Autodesk Fusion 360 part; units mm, degrees
(part 2 of 2)
  arc A185 (36.111, 28.317) -> (36.111, 28.9662) centre (36.111, 28.6416) ccw
  line L756 (10.3187, 51.2288) -> (10.3187, 43.6088)
  line L757 (11.5888, 43.6088) -> (11.5888, 42.8468)
  line L758 (34.6508, 29.4855) -> (34.9754, 29.4855)
  line L759 (34.9754, 28.8363) -> (34.6508, 28.8363)
  arc A186 (9.6537, 49.5828) -> (9.0045, 49.5828) centre (9.3291, 49.5828) ccw
  line L760 (35.4013, 26.035) -> (35.4013, 26.797)
  line L761 (13.335, 43.6088) -> (15.875, 43.6088)
  line L762 (9.5238, 50.7833) -> (9.5238, 50.3938)
  line L763 (13.335, 51.2288) -> (13.335, 43.6088)
  line L764 (14.605, 43.6088) -> (14.605, 42.8468)
  line L765 (15.875, 51.2288) -> (13.335, 51.2288)
  line L766 (10.173, 49.9073) -> (9.6537, 49.6477)
  line L767 (15.875, 43.6088) -> (15.875, 51.2288)
  arc A187 (42.1887, 7.893) -> (41.8275, 7.5318) centre (42.1887, 7.5318) ccw
  line L768 (38.2999, 28.1745) -> (38.0403, 28.6938)
  arc A188 (16.67, 43.5828) -> (16.0208, 43.5828) centre (16.3454, 43.5828) ccw
  line L769 (35.7864, 29.4855) -> (36.1759, 29.4855)
  arc A189 (9.7835, 51.0429) -> (9.5239, 50.7833) centre (9.7835, 50.7833) ccw
  arc A190 (36.1759, 28.9662) -> (36.1759, 29.4854) centre (36.1759, 29.2258) ccw
  arc A191 (37.9754, 28.6938) -> (37.9754, 29.343) centre (37.9754, 29.0184) ccw
  line L770 (36.6713, 26.035) -> (34.1313, 26.035)
  line L771 (12.8588, 51.2288) -> (10.3187, 51.2288)
  arc A192 (34.9754, 28.8363) -> (34.9754, 29.4855) centre (34.9754, 29.1609) ccw
  line L772 (39.5288, 26.035) -> (36.9888, 26.035)
  arc A193 (7.0485, 20.1406) -> (7.6355, 20.2761) centre (7.0485, 21.4802) ccw
  line L773 (9.0926, 39.3417) -> (9.0926, 38.1733)
  line L774 (6.5583, 39.3417) -> (7.2074, 39.3417)
  line L775 (42.3863, 26.035) -> (39.8463, 26.035)
  line L776 (33.492, 39.5042) -> (34.1412, 39.5042)
  arc A194 (40.4754, 28.5513) -> (40.4754, 29.2005) centre (40.4754, 28.8759) ccw
  line L777 (33.8166, 38.3358) -> (33.8166, 39.5042)
  line L778 (41.1163, 18.415) -> (41.1163, 17.653)
  arc A195 (8.8801, 47.012) -> (8.8801, 47.6612) centre (8.8801, 47.3366) ccw
  line L779 (17.1892, 43.2582) -> (16.0208, 43.2582)
  arc A196 (16.7997, 45.0429) -> (16.5401, 44.7833) centre (16.7997, 44.7833) ccw
  line L780 (8.9451, 47.6612) -> (8.6854, 47.6612)
  line L781 (34.6139, 38.3358) -> (34.6139, 39.5042)
  line L782 (8.0047, 38.6926) -> (7.6801, 38.6926)
  arc A197 (16.8646, 44.3938) -> (16.8646, 45.043) centre (16.8646, 44.7184) ccw
  line L783 (40.1508, 28.0321) -> (40.1508, 29.2005)
  line L784 (6.8829, 38.1733) -> (6.8829, 39.3417)
  arc A198 (36.351, 39.2121) -> (36.0589, 39.5042) centre (36.0589, 39.2121) ccw
  arc A199 (7.7922, 47.5313) -> (7.7922, 48.1805) centre (7.7922, 47.8559) ccw
  line L785 (34.9384, 38.8551) -> (34.6139, 38.8551)
  line L786 (41.2864, 29.0706) -> (41.2864, 29.2005)
  line L787 (7.7922, 47.5313) -> (7.4676, 47.5313)
  line L788 (16.6699, 43.5828) -> (16.6699, 43.2582)
  line L789 (36.2536, 38.9849) -> (35.7018, 38.3358)
  line L790 (8.5556, 48.1805) -> (8.9451, 48.1805)
  line L791 (8.7681, 38.1733) -> (9.4172, 38.1733)
  line L792 (10.173, 50.3938) -> (10.173, 50.7833)
  line L793 (7.6801, 39.3417) -> (8.0047, 39.3417)
  line L794 (11.5888, 51.2288) -> (11.5888, 51.9908)
  line L795 (39.8463, 26.035) -> (39.8463, 18.415)
  circle A200 centre (8.0475, 36.6938) radius 1.27
  line L796 (40.1508, 29.2005) -> (40.4754, 29.2005)
  line L797 (42.3863, 18.415) -> (42.3863, 26.035)
  line L798 (39.8463, 18.415) -> (42.3863, 18.415)
  circle A201 centre (8.0412, 45.3738) radius 1.27
  line L799 (6.6704, 47.0121) -> (6.6704, 48.1805)
  line L800 (7.4676, 48.1805) -> (7.7922, 48.1805)
  line L801 (6.3458, 48.1805) -> (6.9949, 48.1805)
  line L802 (40.4754, 28.5513) -> (40.1508, 28.5513)
  arc A202 (8.0047, 38.6925) -> (8.0047, 39.3417) centre (8.0047, 39.0171) ccw
  line L803 (17.1892, 43.9073) -> (16.6699, 43.6477)
  line L804 (41.2864, 29.2005) -> (41.9355, 29.2005)
  line L805 (41.9355, 29.2005) -> (41.611, 28.0321)
  line L806 (8.7681, 39.0821) -> (9.0926, 39.3417)
  line L807 (7.6801, 38.1733) -> (7.6801, 39.3417)
  line L808 (10.173, 49.2582) -> (9.0046, 49.2582)
  line L809 (41.1163, 26.035) -> (41.1163, 26.797)
  arc A203 (16.0208, 44.9131) -> (16.5401, 44.3938) centre (16.5401, 44.9131) ccw
  line L810 (40.7999, 28.0321) -> (40.5403, 28.5513)
  circle A204 centre (35.0288, 36.6975) radius 1.27
  dimension "d1" = 53
  dimension "d2" = 55
  measures "d1" distance of L347 L361
  measures "d2" distance of A48.start A52.end
ref_plane "Arbeitsebene3" through (26.5, 27.5, -3) normal (0, 0, 1) x (1, 0, 0)
sketch "Skizze2" plane through (26.5, 27.5, -3) normal (0, 0, 1) x (1, 0, 0)
  circle A0 centre (-22.5, 23.5) radius 1.5875
  line L0 (25.5, 27.5) -> (-25.5, 27.5)
  arc A1 (-25.5, 27.5) -> (-26.5, 26.5) centre (-25.5, 26.5) ccw
  line L1 (-26.5, -26.5) -> (-26.5, 26.5)
  line L2 (-25.5, -27.5) -> (25.5, -27.5)
  arc A2 (-26.5, -26.5) -> (-25.5, -27.5) centre (-25.5, -26.5) ccw
  arc A3 (25.5, -27.5) -> (26.5, -26.5) centre (25.5, -26.5) ccw
  line L3 (26.5, -26.5) -> (26.5, 26.5)
  arc A4 (26.5, 26.5) -> (25.5, 27.5) centre (25.5, 26.5) ccw
  circle A5 centre (22.5, 23.5) radius 3.1
  circle A6 centre (22.5, 23.5) radius 1.5875
  circle A7 centre (-22.5, 23.5) radius 3.1
  line L4 (-36, -27.5) -> (36, -27.5)
  line L5 (36.5, -27) -> (36.5, 28.5)
  line L6 (34.5, 30.5) -> (-34.5, 30.5)
  line L7 (-36.5, 28.5) -> (-36.5, -27)
  arc A8 (-34.5, 30.5) -> (-36.5, 28.5) centre (-34.5, 28.5) ccw
  arc A9 (36.5, 28.5) -> (34.5, 30.5) centre (34.5, 28.5) ccw
  arc A10 (-36.5, -27) -> (-36, -27.5) centre (-36, -27) ccw
  arc A11 (36, -27.5) -> (36.5, -27) centre (36, -27) ccw
  line L8 (-33.5, -25.5) -> (33.5, -25.5)
  line L9 (34.5, -24.5) -> (34.5, 27.5)
  line L10 (33.5, 28.5) -> (-33.5, 28.5)
  line L11 (-34.5, 27.5) -> (-34.5, -24.5)
  arc A12 (-33.5, 28.5) -> (-34.5, 27.5) centre (-33.5, 27.5) ccw
  arc A13 (-34.5, -24.5) -> (-33.5, -25.5) centre (-33.5, -24.5) ccw
  arc A14 (33.5, -25.5) -> (34.5, -24.5) centre (33.5, -24.5) ccw
  arc A15 (34.5, 27.5) -> (33.5, 28.5) centre (33.5, 27.5) ccw
  line L12 (-27, -25.5) -> (-27, -27.5)
  line L13 (27, -25.5) -> (27, -27.5)
  line L14 (35.3, -24.5) -> (35.3, 27.5)
  arc A16 (35.3, 27.5) -> (33.5, 29.3) centre (33.5, 27.5) ccw
  line L15 (33.5, 29.3) -> (-33.5, 29.3)
  arc A17 (-33.5, 29.3) -> (-35.3, 27.5) centre (-33.5, 27.5) ccw
  line L16 (-35.3, 27.5) -> (-35.3, -24.5)
  arc A18 (-35.3, -24.5) -> (-33.5, -26.3) centre (-33.5, -24.5) ccw
  line L17 (-33.5, -26.3) -> (33.5, -26.3)
  arc A19 (33.5, -26.3) -> (35.3, -24.5) centre (33.5, -24.5) ccw
  circle A20 centre (-22.5, 23.5) radius 4
  circle A21 centre (22.5, 23.5) radius 4
  circle A22 centre (30.75, -19.5) radius 1.75
  circle A23 centre (30.75, -19.5) radius 3.75
  circle A24 centre (-30.75, -19.5) radius 1.75
  circle A25 centre (-30.75, -19.5) radius 3.75
  line L18 (24.5, -5) -> (28.5, -5)
  line L19 (28.5, -5) -> (28.5, -7)
  line L20 (28.5, -7) -> (24.5, -7)
  line L21 (24.5, -7) -> (24.5, -5)
  line L22 (27, -5) -> (27, -7)
  line L23 (-28.5, -5) -> (-24.5, -5)
  line L24 (-24.5, -5) -> (-24.5, -7)
  line L25 (-24.5, -7) -> (-28.5, -7)
  line L26 (-28.5, -7) -> (-28.5, -5)
  line L27 (-27, -5) -> (-27, -7)
  point P0 (-23.84, -27.5)
  point P1 (-26.5, -27.5)
  point P2 (-26.5, -26.5)
  dimension "d6" = 2
  dimension "d7" = 2
  dimension "d8" = 3
  dimension "d9" = 10
  dimension "d10" = 10
  dimension "d11" = 0.5
  dimension "d12" = 0.5
  dimension "d14" = 1
  dimension "d15" = 1
  dimension "d16" = 1
  dimension "d17" = 2
  dimension "d18" = 2
  dimension "d19" = 2
  dimension "d20" = 1
  dimension "d21" = 2
  dimension "d22" = 0.5
  dimension "d23" = 0.5
  dimension "d24" = 0.8
  dimension "d25" = 8
  dimension "d26" = 8
  dimension "d27" = 3.5
  dimension "d28" = 7.5
  dimension "d29" = 3.75
  dimension "d30" = 6
  dimension "d31" = 3.5
  dimension "d32" = 7.5
  dimension "d33" = 3.75
  dimension "d34" = 6
  dimension "d35" = 4
  dimension "d36" = 1.5
  dimension "d37" = 2
  dimension "d38" = 2
  dimension "d39" = 18.5
  dimension "d40" = 2
  dimension "d41" = 4
  dimension "d42" = 18.5
  dimension "d43" = 2
  dimension "d44" = 1.5
  constraint parallel L2 L4
  constraint perpendicular L4 L5
  constraint perpendicular L5 L6
  constraint perpendicular L4 L7
  constraint tangent L6 A8
  constraint tangent L7 A8
  constraint tangent L5 A9
  constraint tangent L6 A9
  constraint collinear L2 L4
  constraint tangent L4 A10
  constraint tangent L7 A10
  constraint tangent L4 A11
  constraint tangent L5 A11
  constraint parallel L4 L8
  constraint parallel L5 L9
  constraint parallel L6 L10
  constraint parallel L7 L11
  constraint tangent L10 A12
  constraint tangent L11 A12
  constraint tangent L8 A13
  constraint tangent L11 A13
  constraint tangent L8 A14
  constraint tangent L9 A14
  constraint tangent L9 A15
  constraint tangent L10 A15
  constraint coincident L8 L12.start
  constraint coincident L4 L12.end
  constraint perpendicular L4 L12
  constraint coincident L8 L13.start
  constraint coincident L4 L13.end
  constraint perpendicular L4 L13
  constraint concentric A7 A20
  constraint concentric A5 A21
  constraint concentric A22 A23
  constraint concentric A24 A25
  constraint horizontal L18
  constraint vertical L19
  constraint horizontal L20
  constraint vertical L21
  constraint coincident L18 L22.start
  constraint coincident L20 L22.end
  constraint perpendicular L20 L22
  constraint horizontal L23
  constraint vertical L24
  constraint horizontal L25
  constraint vertical L26
  constraint coincident L23 L27.start
  constraint coincident L25 L27.end
  constraint perpendicular L25 L27
  measures "d6" radius of A8
  measures "d7" radius of A9
  measures "d8" distance of L0 L6
  measures "d9" distance of L1 L7
  measures "d10" distance of L3 L5
  measures "d11" radius of A10
  measures "d12" radius of A11
  measures "d14" radius of A12
  measures "d15" radius of A13
  measures "d16" radius of A14
  measures "d17" distance of L7 L11
  measures "d18" distance of L6 L10
  measures "d19" distance of L5 L9
  measures "d20" radius of A15
  measures "d21" distance of L4 L8
  measures "d22" distance of L1 L12
  measures "d23" distance of L3 L13
  measures "d25" diameter of A20
  measures "d26" diameter of A21
  measures "d27" diameter of A22
  measures "d28" diameter of A23
  measures "d29" distance of L9 A22.centre
  measures "d30" distance of L8 A22.centre
  measures "d31" diameter of A24
  measures "d32" diameter of A25
  measures "d33" distance of L11 A24.centre
  measures "d34" distance of L8 A24.centre
  measures "d35" distance of L18.start L18.end
  measures "d36" distance of L19.end L22.end
  measures "d37" distance of L18.start L20.end
  measures "d38" distance of L3 L19.end
  measures "d39" distance of L8 L19.end
  measures "d40" distance of L23.end L24.end
  measures "d41" distance of L24.end L25.end
  measures "d42" distance of L8 L25.end
  measures "d43" distance of L1 L23.start
  measures "d44" distance of L26 L27
extrude "Extrusion1" add sketch "Skizze2" against normal blind 2 contours A0 | L0 L3 A4 A21 | A23 | A25 | L0 A1 L1 L3 A4 L8 L9 L10 L11 A12 A13 A14 A15 L18 L19 L20 L23 L25 L26 | L0 L1 L3 L8 A20 A21 L18 L20 L21 L23 L24 L25 | A21 | L0 A1 L1 A20 | A20 | L3 L18 L20 L22 | L3 L18 L20 L21 | L1 L23 L24 L25 | L1 L23 L25 L27 | L18 L19 L20 L22 | L23 L25 L26 L27 | L3 L8 L13 L17 | L1 L3 L8 L17 | L1 L8 L12 L17 | A3 L3 L4 L13 L17 | L1 L2 A2 A3 L3 L4 L17 | L8 L9 L10 L11 A12 A13 A14 A15 L12 L13 L14 A16 L15 A17 L16 A18 L17 A19 | L1 A2 L4 L12 L17 | L4 L5 L6 L7 A8 A9 A10 A11 L12 L13 L14 A16 L15 A17 L16 A18 L17 A19 | A5 | A6 | A7 | A22 | A24 makes body 1
extrude "Extrusion2" add sketch "Skizze2" along normal blind 3 contours A21 | A20 | L3 L18 L20 L22 | L3 L18 L20 L21 | L1 L23 L24 L25 | L1 L23 L25 L27 | L18 L19 L20 L22 | L23 L25 L26 L27 | A5 | A7 bodies 1
chamfer "Fase1" distance 1 angle 45 2 edges at (0.2707, 49.5535, 0) (45.2707, 49.5535, 0) on bodies 1
extrude "Extrusion3" add sketch "Skizze2" along normal blind 4.6 contours L23 L25 L26 L27 bodies 1
extrude "Extrusion4" cut sketch "Skizze2" along normal blind 4.6 contours L18 L19 L20 L22 bodies 1
extrude "Extrusion5" add sketch "Skizze2" along normal blind 4.6 contours L18 L19 L20 L22 bodies 1
extrude "Extrusion6" add sketch "Skizze2" along normal blind 4.6 contours A23 | A25 bodies 1
extrude "Extrusion7" add sketch "Skizze2" along normal blind 2 contours L3 L8 L13 L17 | L1 L3 L8 L17 | L1 L8 L12 L17 | A3 L3 L4 L13 L17 | L1 L2 A2 A3 L3 L4 L17 | L1 A2 L4 L12 L17 bodies 1
extrude "Extrusion8" add sketch "Skizze2" along normal blind 9 contours L4 L5 L6 L7 A8 A9 A10 A11 L12 L13 L14 A16 L15 A17 L16 A18 L17 A19 bodies 1
extrude "Extrusion9" add sketch "Skizze2" along normal blind 10 separate body contours L8 L9 L10 L11 A12 A13 A14 A15 L12 L13 L14 A16 L15 A17 L16 A18 L17 A19 makes body 2
sketch "Skizze3" plane through (0, 0, -5) normal (0, 0, -1) x (1, 0, 0)
  arc A0 (63, -0.5) -> (62.5, 0) centre (62.5, -0.5) ccw
  line L0 (62.5, 0) -> (-9.5, 0)
  arc A1 (-9.5, 0) -> (-10, -0.5) centre (-9.5, -0.5) ccw
  line L1 (-10, -0.5) -> (-10, -56)
  arc A2 (-10, -56) -> (-8, -58) centre (-8, -56) ccw
  line L2 (-8, -58) -> (61, -58)
  arc A3 (61, -58) -> (63, -56) centre (61, -56) ccw
  line L3 (63, -56) -> (63, -0.5)
  circle A4 centre (-4.25, -8) radius 1.75
  circle A5 centre (57.25, -8) radius 1.75
  circle A6 centre (49, -51) radius 1.5875
  circle A7 centre (4, -51) radius 1.5875
  circle A8 centre (-4.25, -8) radius 3
  circle A9 centre (57.25, -8) radius 3
  circle A10 centre (49, -51) radius 3
  circle A11 centre (4, -51) radius 3
  dimension "d64" = 6
  dimension "d65" = 6
  dimension "d66" = 6
  dimension "d67" = 6
  constraint concentric A4 A8
  constraint concentric A5 A9
  constraint concentric A6 A10
  constraint concentric A7 A11
  measures "d64" diameter of A8
  measures "d65" diameter of A9
  measures "d66" diameter of A10
  measures "d67" diameter of A11
extrude "Extrusion10" cut sketch "Skizze3" against normal blind 2 contours A4 | A5 | A6 | A7 bodies 1
extrude "Extrusion11" cut sketch "Skizze3" against normal blind 1.5 contours A8 | A9 | A10 | A11 bodies 1
fillet "Abrundung1" radius 2 8 edges at (-10, 28.25, -5) (-9.4142, 57.4142, -5) (26.5, 58, -5) (62.4142, 57.4142, -5) (63, 28.25, -5) (62.8536, 0.1464, -5) (26.5, 0, -5) (-9.8536, 0.1464, -5) on bodies 1
fillet "Abrundung2" radius 1 4 edges at (0, 22.5, -3) (2, 21.5, -3) (0, 20.5, -3) (-2, 21.5, -3) on bodies 1
fillet "Abrundung3" radius 1 4 edges at (53, 20.5, -3) (51, 21.5, -3) (53, 22.5, -3) (55, 21.5, -3) on bodies 1
combine "Kombinieren1" operation add target body 1 tool bodies 2
ref_plane "Arbeitsebene4" through (26.5, 27.5, 9.6) normal (0, 0, 1) x (1, 0, 0)
sketch "Skizze4" plane through (26.5, 27.5, 9.6) normal (0, 0, 1) x (1, 0, 0)
  line L0 (-36, -27.5) -> (-27, -27.5)
  line L1 (-36.5, 28.5) -> (-36.5, -27)
  arc A0 (-36.5, -27) -> (-36, -27.5) centre (-36, -27) ccw
  arc A1 (-34.5, 30.5) -> (-36.5, 28.5) centre (-34.5, 28.5) ccw
  line L2 (34.5, 30.5) -> (-34.5, 30.5)
  arc A2 (36.5, 28.5) -> (34.5, 30.5) centre (34.5, 28.5) ccw
  line L3 (36.5, -27) -> (36.5, 28.5)
  arc A3 (36, -27.5) -> (36.5, -27) centre (36, -27) ccw
  line L4 (27, -27.5) -> (36, -27.5)
  line L5 (33.5, -25.5) -> (27, -25.5)
  arc A4 (33.5, -25.5) -> (34.5, -24.5) centre (33.5, -24.5) ccw
  line L6 (34.5, 27.5) -> (34.5, -24.5)
  arc A5 (34.5, 27.5) -> (33.5, 28.5) centre (33.5, 27.5) ccw
  line L7 (-33.5, 28.5) -> (33.5, 28.5)
  arc A6 (-33.5, 28.5) -> (-34.5, 27.5) centre (-33.5, 27.5) ccw
  line L8 (-34.5, -24.5) -> (-34.5, 27.5)
  arc A7 (-34.5, -24.5) -> (-33.5, -25.5) centre (-33.5, -24.5) ccw
  line L9 (-27, -25.5) -> (-33.5, -25.5)
  line L10 (27, -25.5) -> (-27, -25.5)
  line L11 (-27, -27.5) -> (27, -27.5)
  line L12 (-26.5, -25.5) -> (-26.5, -27.5)
  line L13 (26.5, -25.5) -> (26.5, -27.5)
  line L14 (27, -26.7) -> (33.7, -26.7)
  line L15 (35.7, -24.7) -> (35.7, 28.5)
  arc A8 (35.7, 28.5) -> (34.5, 29.7) centre (34.5, 28.5) ccw
  line L16 (34.5, 29.7) -> (-34.5, 29.7)
  arc A9 (-34.5, 29.7) -> (-35.7, 28.5) centre (-34.5, 28.5) ccw
  line L17 (-35.7, 28.5) -> (-35.7, -24.7)
  line L18 (-33.7, -26.7) -> (-27, -26.7)
  line L19 (-27, -26.7) -> (-26.5, -26.7)
  line L20 (27, -26.7) -> (26.5, -26.7)
  arc A10 (-35.7, -24.7) -> (-33.7, -26.7) centre (-33.7, -24.7) ccw
  arc A11 (33.7, -26.7) -> (35.7, -24.7) centre (33.7, -24.7) ccw
  line L21 (19.7537, 17.66) -> (26.1038, 17.66)
  line L22 (18.325, 17.66) -> (19.7537, 17.66)
  line L23 (16.8962, 17.66) -> (18.325, 17.66)
  line L24 (16.8962, -2.66) -> (16.8962, 17.66)
  line L25 (26.1038, 17.66) -> (26.1038, 9.5638)
  line L26 (26.1038, 9.5638) -> (26.1038, 5.4362)
  line L27 (26.1038, 5.4362) -> (26.1038, -2.66)
  line L28 (26.1038, -2.66) -> (19.7537, -2.66)
  line L29 (19.7537, -2.66) -> (18.325, -2.66)
  line L30 (18.325, -2.66) -> (16.8962, -2.66)
  line L31 (19.7537, -3.88) -> (26.1038, -3.88)
  line L32 (18.325, -3.88) -> (19.7537, -3.88)
  line L33 (16.8962, -3.88) -> (18.325, -3.88)
  line L34 (16.8962, -19.12) -> (16.8962, -3.88)
  line L35 (18.325, -19.12) -> (16.8962, -19.12)
  line L36 (19.7537, -19.12) -> (18.325, -19.12)
  line L37 (26.1038, -19.12) -> (19.7537, -19.12)
  line L38 (26.1038, -12.77) -> (26.1038, -19.12)
  line L39 (26.1038, -10.23) -> (26.1038, -12.77)
  line L40 (26.1038, -3.88) -> (26.1038, -10.23)
  line L41 (-9.66, 27.1038) -> (-1.5638, 27.1038)
  line L42 (-1.5638, 27.1038) -> (2.5638, 27.1038)
  line L43 (-9.66, 20.7537) -> (-9.66, 27.1038)
  line L44 (-9.66, 19.325) -> (-9.66, 20.7537)
  line L45 (-9.66, 17.8962) -> (-9.66, 19.325)
  line L46 (10.66, 17.8962) -> (-9.66, 17.8962)
  line L47 (10.66, 19.325) -> (10.66, 17.8962)
  line L48 (10.66, 20.7537) -> (10.66, 19.325)
  line L49 (10.66, 27.1038) -> (10.66, 20.7537)
  line L50 (2.5638, 27.1038) -> (10.66, 27.1038)
  line L51 (-10.46, 27.9038) -> (-1.5638, 27.9038)
  line L52 (-1.5638, 27.9038) -> (2.5638, 27.9038)
  line L53 (2.5638, 27.9038) -> (11.46, 27.9038)
  line L54 (11.46, 27.9038) -> (11.46, 20.7537)
  line L55 (11.46, 20.7537) -> (11.46, 19.325)
  line L56 (11.46, 19.325) -> (11.46, 17.0962)
  line L57 (11.46, 17.0962) -> (-10.46, 17.0962)
  line L58 (-10.46, 17.0962) -> (-10.46, 19.325)
  line L59 (-10.46, 19.325) -> (-10.46, 20.7537)
  line L60 (-10.46, 20.7537) -> (-10.46, 27.9038)
  line L61 (16.0962, 18.46) -> (26.9038, 18.46)
  line L62 (26.9038, 18.46) -> (26.9038, -19.92)
  line L63 (26.9038, -19.92) -> (16.0962, -19.92)
  line L64 (16.0962, -19.92) -> (16.0962, 18.46)
  circle A12 centre (22.5, 23.5) radius 1.25
  circle A13 centre (22.5, 23.5) radius 3
  circle A14 centre (-22.5, 23.5) radius 1.25
  circle A15 centre (-22.5, 23.5) radius 3
  circle A16 centre (-30.75, -19.5) radius 1.25
  circle A17 centre (-30.75, -19.5) radius 3
  circle A18 centre (30.75, -19.5) radius 1.25
  circle A19 centre (30.75, -19.5) radius 3
  dimension "d82" = 10
  dimension "d83" = 10
  dimension "d85" = 2
  dimension "d86" = 2
  dimension "d87" = -0.8
  dimension "d88" = 0.8
  dimension "d89" = 0.8
  dimension "d90" = 0.8
  dimension "d91" = 0.8
  dimension "d92" = 2.5
  dimension "d93" = 6
  dimension "d94" = 2.5
  dimension "d95" = 6
  dimension "d96" = 2.5
  dimension "d97" = 6
  dimension "d98" = 2.5
  dimension "d99" = 6
  dimension "d100" = 0.8
  dimension "d101" = 0.8
  dimension "d102" = 0.8
  dimension "d103" = 5.75
  dimension "d104" = 8
  dimension "d105" = 5.75
  dimension "d106" = 8
  constraint coincident L10 L12.start
  constraint coincident L11 L12.end
  constraint perpendicular L11 L12
  constraint coincident L10 L13.start
  constraint coincident L11 L13.end
  constraint perpendicular L11 L13
  constraint coincident L12 L19.end
  constraint perpendicular L12 L19
  constraint coincident L13 L20.end
  constraint perpendicular L13 L20
  constraint parallel L4 L14
  constraint parallel L3 L15
  constraint concentric A2 A8
  constraint parallel L2 L16
  constraint concentric A1 A9
  constraint parallel L1 L17
  constraint parallel L0 L18
  constraint tangent A9 L17
  constraint tangent L15 A8
  constraint tangent A8 L16
  constraint tangent L16 A9
  constraint tangent L17 A10
  constraint tangent L18 A10
  constraint tangent L14 A11
  constraint tangent L15 A11
  constraint horizontal L61
  constraint vertical L62
  constraint horizontal L63
  constraint vertical L64
  constraint concentric A12 A13
  constraint concentric A16 A17
  measures "d82" horizontal distance of L1.end L12.end
  measures "d83" horizontal distance of L3.start L13.end
  measures "d85" radius of A10
  measures "d86" radius of A11
  measures "d88" distance of L34.start L63
  measures "d89" distance of L23.start L61
  measures "d90" distance of L23.start L64
  measures "d91" horizontal distance of L21.end L61.end
  measures "d92" diameter of A12
  measures "d93" diameter of A13
  measures "d94" diameter of A14
  measures "d95" diameter of A15
  measures "d96" diameter of A16
  measures "d97" diameter of A17
  measures "d98" diameter of A18
  measures "d99" diameter of A19
  measures "d100" distance of L3 L15
  measures "d101" distance of L4 L14
  measures "d102" distance of L12.end L19.end
  measures "d103" distance of L1 A16.centre
  measures "d104" distance of L0 A16.centre
  measures "d105" distance of L3 A18.centre
  measures "d106" distance of L4 A18.centre
extrude "Extrusion13" add sketch "Skizze4" along normal blind 2 separate body contours L0 L1 A0 A1 L2 A2 L3 A3 L4 L11 L12 L13 L14 L15 A8 L16 A9 L17 L18 L19 L20 A10 A11 | L10 L11 L12 L13 | L5 A4 L6 A5 L7 A6 L8 A7 L9 L10 L12 L13 L14 L15 A8 L16 A9 L17 L18 L19 L20 A10 A11 | L5 A4 L6 A5 L7 A6 L8 A7 L9 L10 | A12 | A13 | A14 | A15 | A16 | A17 | A18 | A19 makes body 3
extrude "Extrusion14" add sketch "Skizze4" against normal blind 3.4 separate body contours L0 L1 A0 A1 L2 A2 L3 A3 L4 L11 L12 L13 L14 L15 A8 L16 A9 L17 L18 L19 L20 A10 A11 | L10 L11 L12 L13 makes body 4
extrude "Extrusion15" add sketch "Skizze4" against normal blind 2.4 separate body contours L5 A4 L6 A5 L7 A6 L8 A7 L9 L10 L12 L13 L14 L15 A8 L16 A9 L17 L18 L19 L20 A10 A11 makes body 5
extrude "Extrusion16" add sketch "Skizze4" against normal blind 7.7 separate body contours A17 | A19 makes body 6 at (-1.2537, 7.8505, 4.4667) makes body 7 at (60.2463, 7.8505, 4.4667)
extrude "Extrusion17" add sketch "Skizze4" against normal blind 6.1 separate body contours A13 | A15 makes body 8 at (6.9963, 50.8505, 5.5333) makes body 9 at (51.9963, 50.8505, 5.5333)
combine "Kombinieren2" operation add target body 3 tool bodies 4 5 6 7 8 9
fillet "Abrundung4" radius 2 8 edges at (-10, 28.25, 11.6) (-9.8536, 0.1464, 11.6) (26.5, 0, 11.6) (62.8536, 0.1464, 11.6) (63, 28.25, 11.6) (62.4142, 57.4142, 11.6) (26.5, 58, 11.6) (-9.4142, 57.4142, 11.6) on bodies 3
fillet "Abrundung5" radius 0.5 1 edges at (42.5962, 7.58, 10.6) on bodies 3
fillet "Abrundung6" radius 0.5 1 edges at (42.5962, 45.96, 10.6) on bodies 3
fillet "Abrundung7" radius 0.5 1 edges at (53.4038, 7.58, 10.6) on bodies 3
fillet "Abrundung8" radius 0.5 1 edges at (53.4038, 45.96, 10.6) on bodies 3
fillet "Abrundung9" radius 0.5 1 edges at (16.04, 55.4038, 10.6) on bodies 3
fillet "Abrundung10" radius 0.5 3 edges at (37.96, 55.4038, 10.6) (16.04, 44.5962, 10.6) (37.96, 44.5962, 10.6) on bodies 3
equation "d9 = d10"
equation "d29 = d28 / 2"
equation "d33 = d29"
equation "d34 = d30"
equation "d40 = d37"
equation "d41 = d35"
equation "d42 = d39"
equation "d43 = d38"
equation "d44 = d36"
equation "d105 = d103"
equation "d106 = d104"
named bodies: "bottom shell UP", "top shell UP"
